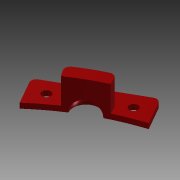
# Autodesk Inventor part: glass clamp
Saved by Autodesk Inventor 2015 SP1 (Build 190203100, 203)
## iProperties
Created: 2015-02-07
Part Number: glass clamp
Material: Generic
Document SubType Name: Modeling
Designer: Joseph
Density: 1 g/cm^3
Appearance: Red
Author: Joseph
Autodesk Inventor part; units mm, degrees
ref_plane "YZ Plane" through (0, 0, 0) normal (1, 0, 0) x (0, 1, 0)
ref_plane "XZ Plane" through (0, 0, 0) normal (0, 1, 0) x (-1, 0, 0)
ref_plane "Work Plane1" through (0, 0, 0) normal (0, 0, 1) x (1, 0, 0)
sketch "Sketch1" plane through (0, 0, 0) normal (0, 0, 1) x (1, 0, 0)
  circle A0 centre (-57.3972, 75.6899) radius 1.7 projected
  circle A1 centre (-35.7169, 88.018) radius 1.7 projected
  line L0 (-64.5902, 76.2012) -> (-59.595, 67.4167)
  line L1 (-32.4784, 94.461) -> (-27.4832, 85.6765)
  line L2 (-63.8402, 78.9284) -> (-35.2055, 95.211)
  circle A2 centre (-57.3972, 75.6899) radius 6 construction
  circle A3 centre (-35.7169, 88.018) radius 6 construction
  arc A4 (-63.8402, 78.9284) -> (-64.5902, 76.2012) centre (-62.8516, 77.1898) ccw
  arc A5 (-32.4784, 94.461) -> (-35.2055, 95.211) centre (-34.2169, 93.4724) ccw
  circle A6 centre (0.0084, -0.0181) radius 121.0993 construction
  line L3 (43.3818, 164.857) -> (-164.4643, 44.857) construction
  line L4 (121.1077, -138.0506) -> (121.1077, 138.0145) construction
  line L5 (-164.4643, -44.8931) -> (43.3818, -164.8931) construction
  circle A7 centre (0.0084, -0.0181) radius 90 construction
  arc A8 (-27.4832, 85.6765) -> (-59.595, 67.4167) centre (-0.044, 0.0559) ccw
  dimension "d4" = 180
  dimension "d0" = 12
  dimension "d1" = 12
  dimension "d2" = 2
  constraints: 11 tangent, 6 centre point, 6 end point, 6 point on circle, 3 coincident, 2 perpendicular, 1 equal radius, 1 parallel, 3 other
  measures "d0" diameter of A2
  measures "d1" diameter of A3
  measures "d2" radius of A4
extrude "Extrusion1" add sketch "Sketch1" along normal blind 2
sketch "Sketch2" plane through (0, 0, 2) normal (0, 0, 1) x (1, 0, 0)
  circle A0 centre (-35.7169, 88.018) radius 1.7 projected
  circle A1 centre (-57.3972, 75.6899) radius 1.7 projected
  arc A2 (-27.4832, 85.6765) -> (-59.595, 67.4167) centre (-0.044, 0.0559) ccw projected
  line L0 (-35.2055, 95.211) -> (-63.8402, 78.9284) projected
  circle A3 centre (-57.3972, 75.6899) radius 5 construction
  circle A4 centre (-35.7169, 88.018) radius 5 construction
  line L1 (-49.5229, 87.0697) -> (-44.487, 78.2135) construction
  line L2 (-52.1804, 76.9063) -> (-50.5205, 74.4596)
  line L3 (-39.4297, 84.1568) -> (-38.1758, 81.4792)
  arc A5 (-42.0496, 85.1378) -> (-51.6839, 79.6594) centre (-19.7869, 34.7758) ccw
  arc A6 (-38.1758, 81.4792) -> (-50.5205, 74.4596) centre (-0.044, 0.0559) ccw
  arc A7 (-51.6839, 79.6594) -> (-52.1804, 76.9063) centre (-50.5253, 78.0291) ccw
  arc A8 (-39.4297, 84.1568) -> (-42.0496, 85.1378) centre (-41.2409, 83.3085) ccw
  point P0 (0, 0)
  point P1 (-53.2595, 78.4969)
  point P2 (-40.2449, 85.8975)
  dimension "d7" = 10
  dimension "d8" = 10
  dimension "d9" = 2
  constraints: 14 point on circle, 6 end point, 4 centre point, 4 tangent, 2 coincident, 2 line through centre, 2 point on line, 1 equal radius, 1 midpoint, 8 other
  measures "d9" radius of A7
extrude "Extrusion2" add sketch "Sketch2" along normal blind 10 contours A2 L2 A7 A5 A8 L3
sketch "Sketch3" plane through (0, 0, 0) normal (0, 0, -1) x (-1, 0, 0)
  arc A0 (59.595, 67.4167) -> (27.4832, 85.6765) centre (0.044, 0.0559) ccw projected
  circle A1 centre (44.487, 78.2135) radius 5
  line L0 (40.1873, 80.7656) -> (48.7866, 75.6615)
  point P0 (0, 0)
  dimension "d12" = 10
  constraints: 3 point on circle, 2 end point, 1 centre point, 1 midpoint
  measures "d12" diameter of A1
revolve "Revolution1" cut sketch "Sketch3" angle 360 about axis through (-40.1873, 80.7656, 0) along (-0.8599304, -0.5104113, 0) picked at (45.5743, 75.9819) picked at (48.3072, 75.9308) picked at (41.5919, 79.8659) contours A1 A0 L0 | A0 L0 A1 | A1 L0 A0
fillet "Fillet1" radius 2 5 edges at (-52.4936, 78.3841, 12) (-47.0049, 82.6416, 12) (-40.5396, 85.1815, 12) (-38.8028, 82.818, 12) (-51.3505, 75.6829, 12)
body "Solid1"
